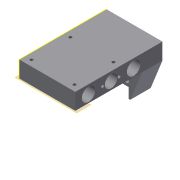
# Autodesk Inventor part: 01_Slide_camera_x_v0
Saved by Autodesk Inventor 2019.4 (Build 234330000, 330)
## iProperties
Created: 2020-10-27
Part Number: 01_Slide_camera_x_v0
Material: Generic
Document SubType Name: Modeling
Designer: diederichbenedict
Density: 1 g/cm^3
Appearance: Default
Author: diederichbenedict
Autodesk Inventor part; units mm, degrees
ref_plane "YZ Plane" through (0, 0, 0) normal (1, 0, 0) x (0, 1, 0)
ref_plane "XZ Plane" through (0, 0, 0) normal (0, 1, 0) x (-1, 0, 0)
ref_plane "XY Plane" through (0, 0, 0) normal (0, 0, 1) x (1, 0, 0)
ref_plane "Work Plane5" through (13.4046, 50.1721, 72.2727) normal (0, 1, 0) x (1, 0, 0)
sketch "Sketch7" plane through (13.4046, 50.1721, 72.2727) normal (0, 1, 0) x (1, 0, 0)
  circle A0 centre (6.5, 6.5) radius 2.5 construction
  circle A1 centre (48.5, 6.5) radius 2.5 construction
  line L0 (55, 2) -> (55, 11) construction
  line L1 (55, 35) -> (55, 44) construction
  circle A2 centre (48.5, 39.5) radius 2.5 construction
  circle A3 centre (6.5, 39.5) radius 2.5 construction
  line L2 (0, 35) -> (0, 44) construction
  line L3 (16.5, 85.8) -> (16.5, 84) construction
  line L4 (38.5, 85.8) -> (38.5, 84) construction
  line L5 (38.5, 84) -> (16.5, 84) construction
  line L6 (2, 0) -> (53, 0) construction
  line L7 (0, 0.7299) -> (55, 0.7299)
  line L8 (55, 0.7299) -> (55, 85.8)
  line L9 (55, 85.8) -> (0, 85.8)
  line L10 (0, 85.8) -> (0, 0.7299)
  point P0 (-13.4046, 72.2727)
  constraints: 22 end point, 5 vertical, 4 centre point, 3 horizontal, 2 parallel, 1 perpendicular, 1 point on line, 20 other
extrude "Extrusion7" add sketch "Sketch7" along normal blind 16
sketch "Sketch8" plane through (13.4046, 50.1721, -13.5273) normal (-1, 0, 0) x (0, 0, 1)
  circle A0 centre (50.2042, 7.5) radius 4
  circle A1 centre (72.2042, 7.5) radius 4
  circle A2 centre (28.2042, 7.5) radius 4
  circle A3 centre (50.2042, 7.5) radius 6
  circle A4 centre (72.2042, 7.5) radius 6
  circle A5 centre (72.2042, 7.5) radius 6.5
  circle A6 centre (28.2042, 7.5) radius 6
  circle A7 centre (28.2042, 7.5) radius 6.5
  point P0 (13.5273, -50.1721)
  dimension "d35" = 8
  dimension "d36" = 8
  dimension "d37" = 0
  dimension "d38" = 22
  dimension "d39" = 22
  dimension "d40" = 12
  dimension "d61" = 0.5
  dimension "d62" = 0.5
  constraints: 8 centre point, 1 coincident, 6 other
  measures "d35" diameter of A1
  measures "d36" diameter of A2
  measures "d37" vertical distance of A1.centre A0.centre
  measures "d38" distance of A0.centre A1.centre
  measures "d39" distance of A2.centre A0.centre
  measures "d40" diameter of A3
  measures "d61" radial gap between concentric circles of A4 A5
  measures "d62" radial gap between concentric circles of A6 A7
extrude "Extrusion8" cut sketch "Sketch8" against normal through all contours A0 | A1 | A2 | A3 | A4 | A5 | A6 | A7
sketch "Sketch9" plane through (13.4046, 50.1721, 72.2727) normal (0, -1, 0) x (1, 0, 0)
  circle A0 centre (6.5, -6.5) radius 2.5
  circle A1 centre (48.5, -6.5) radius 2.5
  circle A2 centre (48.5, -44.5) radius 2.5
  line L0 (4.5, -51) -> (4.5, 149)
  circle A3 centre (6.5, -44.5) radius 2.5
  point P0 (-13.4046, -72.2727)
  constraints: 4 centre point, 2 end point, 1 vertical, 10 other
hole "Hole1" at (19.9046, 50.1721, 65.7727) at (61.9046, 50.1721, 65.7727) at (61.9046, 50.1721, 27.7727) at (19.9046, 50.1721, 27.7727) direction (0, 1, 0) diameter 2.9 end through all
sketch "Sketch10" plane through (68.4046, 50.1721, -13.5273) normal (0, 0, -1) x (-1, 0, 0)
  circle A0 centre (39, -26) radius 1
  circle A1 centre (16, -26) radius 1
  circle A2 centre (16, -3) radius 1
  circle A3 centre (39, -3) radius 1.1
  circle A4 centre (27.5, -14.5) radius 12
  circle A5 centre (27.5, -14.5) radius 10.8
  line L0 (55, 0) -> (0, 0) projected
  line L1 (11.5, -29) -> (43.5, -29)
  line L2 (43.5, -29) -> (43.5, 0)
  line L3 (43.5, 0) -> (11.5, 0)
  line L4 (11.5, 0) -> (11.5, -29)
  line L5 (11.5, -29) -> (43.5, 0) construction
  line L6 (43.5, -29) -> (11.5, 0) construction
  line L7 (0, 0) -> (11.5, 0)
  line L8 (43.5, 0) -> (55, 0)
  line L9 (55, 0) -> (43.5, 0)
  line L10 (43.5, 0) -> (43.5, -29)
  line L11 (43.5, -29) -> (55, -29)
  line L12 (55, -29) -> (55, 0)
  line L13 (11.5, -29) -> (0, -29)
  line L14 (0, -29) -> (0, 0)
  line L15 (0, 0) -> (11.5, 0)
  line L16 (11.5, 0) -> (11.5, -29)
  circle A6 centre (47.5, -14.5) radius 3 construction
  circle A7 centre (7.5, -14.5) radius 3 construction
  circle A8 centre (47.5, -14.5) radius 3.1
  circle A9 centre (7.5, -14.5) radius 3.1
  point P0 (68.4046, -50.1721)
  dimension "d50" = 24
  dimension "d51" = 32
  dimension "d67" = 6.2
  dimension "d68" = 6.2
  constraints: 32 end point, 10 centre point, 6 parallel, 3 horizontal, 3 perpendicular, 2 coincident, 2 collinear, 2 midpoint, 1 point on line, 14 other
  measures "d50" diameter of A4
  measures "d51" distance of L3.end L2.end
  measures "d67" diameter of A8
  measures "d68" diameter of A9
extrude "Extrusion9" add sketch "Sketch10" against normal blind 10 contours L12 L11 L2 L0 | L2 L1 L4 L0 | L4 L13 L14 L0
sketch "Sketch11" plane through (13.4046, 50.1721, 71.5428) normal (-1, 0, 0) x (0, 0, 1)
  circle A0 centre (-34.8659, 7.5) radius 11
  line L0 (-75.0701, 0) -> (0, 0) projected
  line L1 (-26.8191, 0) -> (-42.9126, 0)
  line L2 (0, 16) -> (-85.0701, 16) projected
  line L3 (-41.848, 16) -> (-27.8837, 16)
  circle A1 centre (-34.8659, 7.5) radius 11
  circle A2 centre (-26.8659, 7.5) radius 1.625
  circle A3 centre (-42.8659, 7.5) radius 1.625
  point P0 (-71.5428, -50.1721)
  constraints: 4 centre point, 4 end point, 4 point on circle, 4 point on line, 8 other
hole "Hole2" at (13.4046, 57.6721, 44.6769) at (13.4046, 57.6721, 28.6769) direction (1, 0, 0) diameter 2.9 end through all
ref_plane "Work Plane6" through (68.4046, 66.1721, -83.5273) normal (0, 0, -1) x (-1, 0, 0)
ref_plane "Work Plane7" through (68.4046, 66.1721, 56.4727) normal (0, 0, -1) x (-1, 0, 0)
sketch "Sketch14" plane through (68.4046, 66.1721, 56.4727) normal (0, 0, -1) x (-1, 0, 0)
  circle A0 centre (27.5, -30.5) radius 12 projected
  circle A1 centre (39, -19) radius 1.1 projected
  circle A2 centre (16, -19) radius 1 projected
  circle A3 centre (16, -42) radius 1 projected
  circle A4 centre (39, -42) radius 1 projected
  circle A5 centre (47.5, -30.5) radius 3.1 projected
  circle A6 centre (7.5, -30.5) radius 3.1 projected
  line L0 (55, -45) -> (0, -45) projected
  line L1 (0, -45) -> (0, -16) projected
  line L2 (55, -16) -> (0, -16) projected
  line L3 (55, -16) -> (55, -45) projected
  point P0 (68.4046, -66.1721)
extrude "Extrusion11" add sketch "Sketch14" along normal blind 10 contours A1 | A2 | A3 | A4 | L0 L1 L2 L3
body "Solid2"
